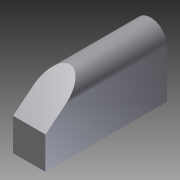
# Autodesk Inventor part: tensioning wedge
Saved by Autodesk Inventor 2012 (Build 160160000, 160)
## iProperties
Created: 2013-07-31
Part Number: tensioning wedge
Material: Default
Document SubType Name: Modeling
Designer: Bryce
Density: 1 g/cm^3
Author: Bryce
Autodesk Inventor part; units mm, degrees
ref_plane "YZ Plane" through (0, 0, 0) normal (1, 0, 0) x (0, 1, 0)
ref_plane "XZ Plane" through (0, 0, 0) normal (0, 1, 0) x (-1, 0, 0)
ref_plane "XY Plane" through (0, 0, 0) normal (0, 0, 1) x (1, 0, 0)
sketch "Sketch1" plane through (0, 0, 0) normal (0, 0, 1) x (1, 0, 0)
  line L0 (0, 0) -> (5.08, 0)
  line L1 (5.08, 0) -> (5.08, 7.62)
  line L2 (0, 7.62) -> (0, 0)
  arc A0 (5.08, 7.62) -> (0, 7.62) centre (2.54, 7.62) ccw
  dimension "d0" = 5.08
  dimension "d1" = 7.62
  constraints: 6 end point, 2 point on circle, 2 tangent, 1 centre point, 1 horizontal, 1 parallel, 1 perpendicular
  measures "d0" distance of L0.start L0.end
  measures "d1" distance of L2.start L0.start
extrude "Extrusion1" add sketch "Sketch1" along normal blind 19.05
sketch "Sketch2" plane through (5.08, 0, 0) normal (1, 0, 0) x (0, 0, -1)
  line L0 (-19.05, 7.62) -> (-19.05, 0) projected
  line L1 (0, 0) -> (0, 7.62) projected
  line L2 (0, 7.62) -> (-19.05, 7.62) projected
  line L3 (0, 7.62) -> (0, 10.16)
  line L4 (0, 10.16) -> (-12.7, 10.16)
  line L5 (-12.7, 10.16) -> (-19.05, 5.08)
  line L6 (-19.05, 5.08) -> (-19.05, 10.16)
  line L7 (-19.05, 10.16) -> (-12.7, 10.16)
  dimension "d4" = 12.7
  dimension "d5" = 5.08
  dimension "d6" = 2.54
  constraints: 10 end point, 4 perpendicular, 1 point on line
  measures "d4" distance from line of L1 L4.end
  measures "d5" distance of L0.end L5.end
  measures "d6" distance between parallel lines of L2 L4
extrude "Extrusion2" cut sketch "Sketch2" against normal through all contours L2 L5 L0 | L6 L7 L5 L2
body "Solid1"
